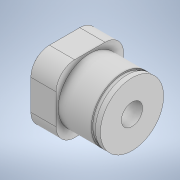
# Autodesk Inventor part: banebot_hubs_large_8mm
Saved by Autodesk Inventor 2020 (Build 240168000, 168)
## iProperties
Created: 2020-02-10
Part Number: banebot_hubs_large_8mm
Material: Generic
Document SubType Name: Modeling
Designer: akend
Density: 1 g/cm^3
Appearance: Default
Author: akend
## iProperties of the stored document _3DPrint.ipt
Created: 2020-02-10
Part Number: _3DPrint
Material: Generic
Document SubType Name: Modeling
Designer: akend
Density: 1 g/cm^3
Appearance: Default
Author: akend
Autodesk Inventor part; units mm, degrees
ref_plane "YZ Plane" through (0, 0, 0) normal (1, 0, 0) x (0, 1, 0)
ref_plane "XZ Plane" through (0, 0, 0) normal (0, 1, 0) x (-1, 0, 0)
ref_plane "XY Plane" through (0, 0, 0) normal (0, 0, 1) x (1, 0, 0)
sketch "Sketch1" plane through (0, 0, 0) normal (1, 0, 0) x (0, 1, 0)
  line L0 (0, 0) -> (20.32, 0)
  line L1 (20.32, 0) -> (20.32, 20.32)
  line L2 (20.32, 20.32) -> (0, 20.32)
  line L3 (0, 20.32) -> (0, 0)
  dimension "d0" = 20.32
  dimension "d1" = 20.32
  constraints: 8 end point, 2 parallel, 1 horizontal, 1 perpendicular
  measures "d0" distance of L2.end L1.end
  measures "d1" distance of L1.end L0.end
extrude "Extrusion1" add sketch "Sketch1" along normal blind 7.62
sketch "Sketch2" plane through (7.62, 0, 0) normal (1, 0, 0) x (0, 0, -1)
  circle A0 centre (-10.16, 10.16) radius 9.525
  point P0 (0, 0)
  dimension "d4" = 19.05
  constraints: 1 centre point
  measures "d4" diameter of A0
extrude "Extrusion2" add sketch "Sketch2" along normal blind 12.7
fillet "Fillet1" radius 5.588 4 edges at (3.81, 20.32, 0) (3.81, 0, 0) (3.81, 0, 20.32) (3.81, 20.32, 20.32)
sketch "Sketch3" plane through (20.32, 10.16, 10.16) normal (1, 0, 0) x (0, 0, -1)
  circle A0 centre (0, 0) radius 9.525
  circle A1 centre (0, 0) radius 9.125
  point P0 (10.16, -10.16)
  dimension "d8" = 18.25
  constraints: 2 centre point, 1 coincident
  measures "d8" diameter of A1
extrude "Extrusion3" cut sketch "Sketch3" against normal blind 2.72
sketch "Sketch4" plane through (20.32, 10.16, 10.16) normal (1, 0, 0) x (0, 0, -1)
  circle A0 centre (0, 0) radius 9.525
  point P0 (10.16, -10.16)
  constraints: 1 centre point
extrude "Extrusion4" add sketch "Sketch4" against normal blind 1.5
sketch "Sketch5" plane through (0, 0, 0) normal (-1, 0, 0) x (0, 0, 1)
  circle A0 centre (10.16, 10.16) radius 9.125 projected
  circle A1 centre (10.16, 10.16) radius 4
  point P0 (0, 0)
  dimension "d13" = 8
  constraints: 1 centre point, 1 coincident
  measures "d13" diameter of A1
extrude "Extrusion5" cut sketch "Sketch5" against normal blind 25 contours A1
sketch "Sketch6" plane through (0, 0, 0) normal (-1, 0, 0) x (0, 0, 1)
  circle A0 centre (10.16, 10.16) radius 4 projected
  circle A1 centre (10.16, 10.16) radius 4
  circle A2 centre (10.16, 10.16) radius 5
  point P0 (0, 0)
  dimension "d16" = 10
  constraints: 2 centre point, 2 coincident
  measures "d16" diameter of A2
extrude "Extrusion6" add sketch "Sketch6" along normal blind 5
fillet "Fillet2" radius 2 1 edges at (0, 10.16, 5.16)
sketch "Sketch7" plane through (20.32, 10.16, 10.16) normal (1, 0, 0) x (0, 0, -1)
  circle A0 centre (0, 0) radius 4 projected
  circle A1 centre (0, 0) radius 4
  circle A2 centre (0, 0) radius 3.2
  point P0 (10.16, -10.16)
  dimension "d20" = 6.4
  constraints: 2 centre point, 2 coincident
  measures "d20" diameter of A2
extrude "Extrusion7" add sketch "Sketch7" against normal blind 25.32
body "Solid1"
